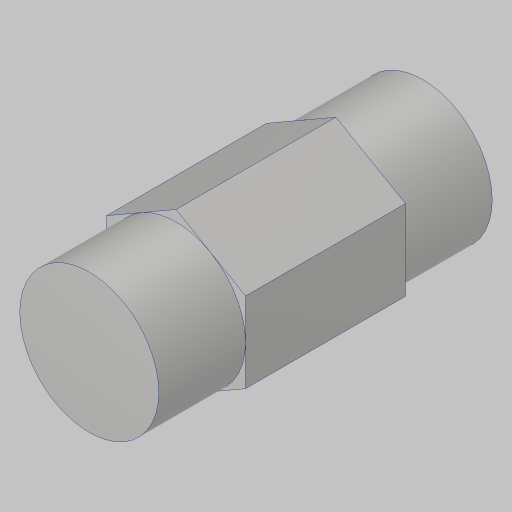
# Autodesk Inventor part: EL2-CGB-011
Saved by Autodesk Inventor 2023.5 (Build 275446000, 446)
## iProperties
RuleStatus: InUse
Created: 2025-01-25
Part Number: EL2-CGB-011
Material: Aluminum 6061
Document SubType Name: Modeling
Designer: brand
Mass: 24.5797 g
Surface Area: 31.4663 cm^2
Volume: 9.10358 cm^3
Density: 2.7 g/cm^3
Appearance: Aluminum - Flat
BeforeDocSave0: size
AfterMaterialChange0: size
AfterFeatureSuppressionChange0: size
PartBodyChanged0: size
AfterDocNew0: SHOW
AfterDocOpen0: SHOW
AfterDocOpen1: size
Author: brand
Autodesk Inventor part; units mm, degrees
ref_plane "YZ Plane" through (0, 0, 0) normal (1, 0, 0) x (0, 1, 0)
ref_plane "XZ Plane" through (0, 0, 0) normal (0, 1, 0) x (-1, 0, 0)
ref_plane "XY Plane" through (0, 0, 0) normal (0, 0, 1) x (1, 0, 0)
sketch "Sketch1" plane through (0, 0, 0) normal (0, 0, 1) x (1, 0, 0)
  line L0 (-6.35, -3.6662) -> (-6.35, 3.6662)
  line L1 (-6.35, 3.6662) -> (0, 7.3323)
  line L2 (0, 7.3323) -> (6.35, 3.6662)
  line L3 (6.35, 3.6662) -> (6.35, -3.6662)
  line L4 (6.35, -3.6662) -> (0, -7.3323)
  line L5 (0, -7.3323) -> (-6.35, -3.6662)
  point P0 (0, 0)
  point P1 (0, 0)
  dimension "Size" = 12.7
  constraints: 12 end point, 1 coincident, 1 vertical alignment, 13 other
  measures "Size" distance between parallel lines of L3 L0
extrude "Extrusion1" add sketch "Sketch1" along normal mid plane 14.6114
sketch "Sketch2" plane through (0, 0, 7.3057) normal (0, 0, 1) x (1, 0, 0)
  line L0 (-6.35, 3.6662) -> (-6.35, -3.6662) construction
  line L1 (-6.35, -3.6662) -> (0, -7.3323) construction
  line L2 (0, -7.3323) -> (6.35, -3.6662) construction
  line L3 (6.35, -3.6662) -> (6.35, 3.6662) construction
  line L4 (6.35, 3.6662) -> (0, 7.3323) construction
  line L5 (0, 7.3323) -> (-6.35, 3.6662) construction
  circle A0 centre (0, 0) radius 6.35
  constraints: 1 centre point, 1 coincident, 1 tangent
extrude "Extrusion2" add sketch "Sketch2" along normal blind 7.9248
mirror "Mirror1" about plane through (0, 0, 0) normal (0, 0, 1) of "Extrusion2"
body "Solid1"
